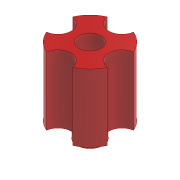
# Autodesk Inventor part: wheel spacer for bearing
Saved by Autodesk Inventor 2020 (Build 240168000, 168)
## iProperties
Created: 2020-02-25
Part Number: wheel spacer for bearing
Material: Generic
Document SubType Name: Modeling
Designer: ball
Density: 1 g/cm^3
Appearance: Default
Author: ball
Autodesk Inventor part; units mm, degrees
ref_plane "YZ Plane" through (0, 0, 0) normal (1, 0, 0) x (0, 1, 0)
ref_plane "XZ Plane" through (0, 0, 0) normal (0, 1, 0) x (-1, 0, 0)
ref_plane "XY Plane" through (0, 0, 0) normal (0, 0, 1) x (1, 0, 0)
sketch "Sketch1" plane through (0, 0, 0) normal (0, 1, 0) x (-1, 0, 0)
  circle A0 centre (0, 0) radius 4.25
  circle A1 centre (0, 0) radius 5
  dimension "d0" = 8.5
  dimension "d1" = 10
  constraints: 3 coincident, 2 centre point
  measures "d0" diameter of A0
  measures "d1" diameter of A1
extrude "Extrusion1" add sketch "Sketch1" along normal blind 31.877
sketch "Sketch2" plane through (0, 31.877, 0) normal (0, 1, 0) x (1, 0, 0)
  circle A0 centre (0, 0) radius 4.25 projected
  arc A1 (5.0369, -11.6585) -> (-5.0369, -11.6585) centre (0, -12.319) ccw
  arc A2 (11.6585, 5.0369) -> (11.6585, -5.0369) centre (12.319, 0) ccw
  arc A3 (-5.0369, 11.6585) -> (5.0369, 11.6585) centre (0, 12.319) ccw
  arc A4 (-11.6585, -5.0369) -> (-11.6585, 5.0369) centre (-12.319, 0) ccw
  arc A5 (-11.6585, -5.0369) -> (-5.0369, -11.6585) centre (0, 0) ccw
  arc A6 (-5.0369, 11.6585) -> (-11.6585, 5.0369) centre (0, 0) ccw
  arc A7 (5.0369, -11.6585) -> (11.6585, -5.0369) centre (0, 0) ccw
  arc A8 (11.6585, 5.0369) -> (5.0369, 11.6585) centre (0, 0) ccw
  circle A9 centre (0, 0) radius 4.25
  dimension "d5" = 10.16
  dimension "d6" = 12.319
  dimension "d9" = 360
  constraints: 16 point on circle, 9 centre point, 2 coincident, 1 concentric, 17 other
  measures "d5" diameter of A1
  measures "d6" distance of point (0, 0) A1.centre
extrude "Extrusion2" add sketch "Sketch2" against normal blind 26.0096
body "Solid1"
